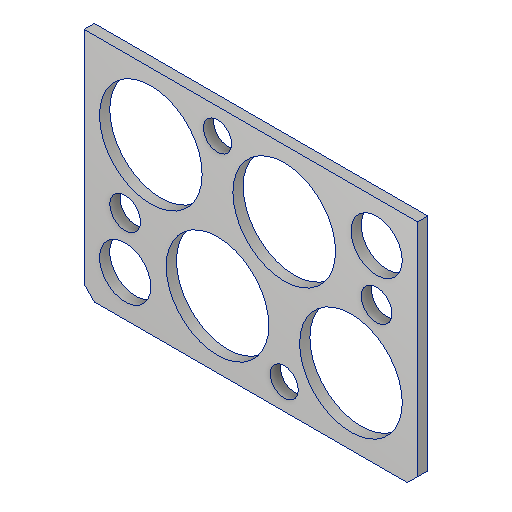
# Autodesk Inventor part: CNCM_ALU_First_sieve
Saved by Autodesk Inventor 2025 (Build 290162010, 162A)
## iProperties
Created: 2018-09-12
Part Number: CNCM_ALU_First_sieve
Material: Aluminum 6061
Document SubType Name: Modeling
Designer: Andrzej
Density: 2.7 g/cm^3
Appearance: Aluminum - Flat
Mass: 7.57738 g
Surface Area: 40.1458 cm^2
Volume: 2.80644 cm^3
Author: Andrzej
Autodesk Inventor part; units mm, degrees
ref_plane "YZ Plane" through (0, 0, 0) normal (1, 0, 0) x (0, 1, 0)
ref_plane "XZ Plane" through (0, 0, 0) normal (0, 1, 0) x (-1, 0, 0)
ref_plane "XY Plane" through (0, 0, 0) normal (0, 0, 1) x (1, 0, 0)
sketch "Sketch1" plane through (0, 0, 0) normal (0, 0, 1) x (1, 0, 0)
  line L0 (-48.3526, 6.9347) -> (16.6474, 6.9347)
  line L1 (16.6474, 6.9347) -> (16.6474, -38.0653)
  line L2 (16.6474, -38.0653) -> (-48.3526, -38.0653)
  line L3 (-48.3526, -38.0653) -> (-48.3526, 6.9347)
  circle A0 centre (-35.3526, -6.0653) radius 10
  circle A1 centre (-22.3526, -25.0653) radius 10
  circle A2 centre (-9.3526, -6.0653) radius 10
  circle A3 centre (3.6474, -25.0653) radius 10
  circle A4 centre (-40.3526, -30.0653) radius 5
  circle A5 centre (8.6474, -1.0653) radius 5
  circle A6 centre (-40.3526, -20.0653) radius 3
  circle A7 centre (8.6474, -11.0653) radius 3
  circle A8 centre (-9.3526, -33.0653) radius 2.75
  circle A9 centre (-22.3526, 1.9347) radius 2.75
  dimension "d1" = 65
  dimension "d2" = 45
  dimension "d3" = 20
  dimension "d10" = 13
  dimension "d11" = 13
  dimension "d40" = 20
  dimension "d41" = 20
  dimension "d42" = 20
  dimension "d43" = 13
  dimension "d44" = 13
  dimension "d45" = 39
  dimension "d46" = 39
  dimension "d47" = 10
  dimension "d48" = 10
  dimension "d49" = 8
  dimension "d50" = 8
  dimension "d51" = 8
  dimension "d52" = 8
  dimension "d53" = 6
  dimension "d54" = 6
  dimension "d55" = 18
  dimension "d56" = 18
  dimension "d57" = 5.5
  dimension "d58" = 5.5
  dimension "d59" = 5
  dimension "d60" = 5
  constraints: 10 centre point, 8 end point, 2 horizontal alignment, 2 parallel, 1 horizontal, 1 perpendicular
  measures "d1" distance of L0.start L0.end
  measures "d2" distance of L0.end L1.end
  measures "d3" diameter of A0
  measures "d10" distance from line of L3 A0.centre
  measures "d11" distance from line of L0 A0.centre
  measures "d40" diameter of A1
  measures "d41" diameter of A2
  measures "d42" diameter of A3
  measures "d43" distance from line of L2 A3.centre
  measures "d44" distance from line of L1 A3.centre
  measures "d45" distance from line of L1 A1.centre
  measures "d46" distance from line of L3 A2.centre
  measures "d47" diameter of A4
  measures "d48" diameter of A5
  measures "d49" distance from line of L1 A5.centre
  measures "d50" distance from line of L3 A4.centre
  measures "d51" distance from line of L2 A4.centre
  measures "d52" distance from line of L0 A5.centre
  measures "d53" diameter of A6
  measures "d54" diameter of A7
  measures "d55" distance from line of L2 A6.centre
  measures "d56" distance from line of L0 A7.centre
  measures "d57" diameter of A8
  measures "d58" diameter of A9
  measures "d59" distance from line of L0 A9.centre
  measures "d60" distance from line of L2 A8.centre
extrude "Extrusion1" add sketch "Sketch1" along normal blind 2
chamfer "Chamfer2" distance 2 angle 45 2 edges at (-48.3526, -38.0653, 1) (16.6474, -38.0653, 1)
equation "\"d10\" = d11"
equation "\"d40\" = d3"
equation "\"d41\" = d3"
equation "\"d42\" = d3"
equation "\"d43\" = d11"
equation "\"d44\" = d11"
body "Solid1"
